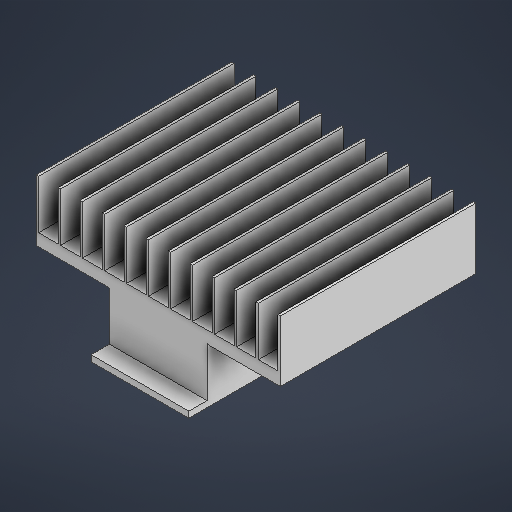
# Autodesk Inventor part: Heatsink_and_Amplifier
Saved by Autodesk Inventor 2026.2 (Build 302298010, 298A)
## iProperties
Created: 2026-09-21
Part Number: Heatsink_and_Amplifier
Material: Generic
Document SubType Name: Modeling
Designer: aiden
Density: 1 g/cm^3
Appearance: Default
Author: aiden
Autodesk Inventor part; units mm, degrees
ref_plane "YZ Plane" through (0, 0, 0) normal (1, 0, 0) x (0, 1, 0)
ref_plane "XZ Plane" through (0, 0, 0) normal (0, 1, 0) x (-1, 0, 0)
ref_plane "XY Plane" through (0, 0, 0) normal (0, 0, 1) x (1, 0, 0)
sketch "Sketch1" plane through (0, 0, 0) normal (0, 1, 0) x (-1, 0, 0)
  line L0 (-63.5, -50.8) -> (63.5, -50.8)
  line L1 (63.5, -50.8) -> (63.5, 50.8)
  line L2 (63.5, 50.8) -> (-63.5, 50.8)
  line L3 (-63.5, 50.8) -> (-63.5, -50.8)
  line L4 (-63.5, -50.8) -> (63.5, 50.8) construction
  line L5 (63.5, -50.8) -> (-63.5, 50.8) construction
  point P0 (0, 0)
  dimension "d0" = 127
  dimension "d1" = 101.6
  constraints: 12 end point, 2 midpoint, 2 parallel, 1 horizontal, 1 perpendicular
  measures "d0" distance of L2.end L1.end
  measures "d1" distance of L1.end L0.end
extrude "Extrusion1" add sketch "Sketch1" along normal blind 31.75
sketch "Sketch2" plane through (-63.5, 0, 50.8) normal (0, 0, 1) x (1, 0, 0)
  line L0 (0, 0) -> (127, 0) projected
  line L1 (0, 0) -> (0, 6.35)
  line L2 (0, 31.75) -> (127, 31.75) projected
  line L3 (0, 6.35) -> (127, 6.35) construction
  line L4 (127, 0) -> (0, 0)
  line L5 (0, 6.35) -> (0, 31.75)
  line L6 (0, 31.75) -> (1.27, 31.75)
  line L7 (1.27, 31.75) -> (1.27, 6.35)
  line L8 (1.27, 6.35) -> (0, 6.35)
  line L9 (127, 0) -> (127, 31.75) projected
  line L10 (127, 31.75) -> (127, 0)
  line L11 (11.43, 6.35) -> (11.43, 31.75)
  line L12 (11.43, 31.75) -> (12.7, 31.75)
  line L13 (12.7, 31.75) -> (12.7, 6.35)
  line L14 (12.7, 6.35) -> (11.43, 6.35)
  line L15 (22.86, 6.35) -> (22.86, 31.75)
  line L16 (22.86, 31.75) -> (24.13, 31.75)
  line L17 (24.13, 31.75) -> (24.13, 6.35)
  line L18 (24.13, 6.35) -> (22.86, 6.35)
  line L19 (34.29, 6.35) -> (34.29, 31.75)
  line L20 (34.29, 31.75) -> (35.56, 31.75)
  line L21 (35.56, 31.75) -> (35.56, 6.35)
  line L22 (35.56, 6.35) -> (34.29, 6.35)
  line L23 (45.72, 6.35) -> (45.72, 31.75)
  line L24 (45.72, 31.75) -> (46.99, 31.75)
  line L25 (46.99, 31.75) -> (46.99, 6.35)
  line L26 (46.99, 6.35) -> (45.72, 6.35)
  line L27 (57.15, 6.35) -> (57.15, 31.75)
  line L28 (57.15, 31.75) -> (58.42, 31.75)
  line L29 (58.42, 31.75) -> (58.42, 6.35)
  line L30 (58.42, 6.35) -> (57.15, 6.35)
  line L31 (68.58, 6.35) -> (68.58, 31.75)
  line L32 (68.58, 31.75) -> (69.85, 31.75)
  line L33 (69.85, 31.75) -> (69.85, 6.35)
  line L34 (69.85, 6.35) -> (68.58, 6.35)
  line L35 (80.01, 6.35) -> (80.01, 31.75)
  line L36 (80.01, 31.75) -> (81.28, 31.75)
  line L37 (81.28, 31.75) -> (81.28, 6.35)
  line L38 (81.28, 6.35) -> (80.01, 6.35)
  line L39 (91.44, 6.35) -> (91.44, 31.75)
  line L40 (91.44, 31.75) -> (92.71, 31.75)
  line L41 (92.71, 31.75) -> (92.71, 6.35)
  line L42 (92.71, 6.35) -> (91.44, 6.35)
  line L43 (102.87, 6.35) -> (102.87, 31.75)
  line L44 (102.87, 31.75) -> (104.14, 31.75)
  line L45 (104.14, 31.75) -> (104.14, 6.35)
  line L46 (104.14, 6.35) -> (102.87, 6.35)
  line L47 (114.3, 6.35) -> (114.3, 31.75)
  line L48 (114.3, 31.75) -> (115.57, 31.75)
  line L49 (115.57, 31.75) -> (115.57, 6.35)
  line L50 (115.57, 6.35) -> (114.3, 6.35)
  line L51 (125.73, 6.35) -> (125.73, 31.75)
  line L52 (125.73, 31.75) -> (127, 31.75)
  line L53 (127, 31.75) -> (127, 6.35)
  line L54 (127, 6.35) -> (125.73, 6.35)
  line L55 (0, 31.75) -> (127, 31.75)
  line L56 (127, 31.75) -> (127, 6.35)
  line L57 (127, 6.35) -> (0, 6.35)
  line L58 (0, 6.35) -> (0, 31.75)
  point P0 (0.635, 31.75)
  point P1 (12.065, 31.75)
  point P2 (23.495, 31.75)
  point P3 (34.925, 31.75)
  point P4 (46.355, 31.75)
  point P5 (57.785, 31.75)
  point P6 (69.215, 31.75)
  point P7 (80.645, 31.75)
  point P8 (92.075, 31.75)
  point P9 (103.505, 31.75)
  point P10 (114.935, 31.75)
  point P11 (126.365, 31.75)
  point P12 (126.365, 31.75)
  point P13 (125.73, 6.35)
  point P14 (115.57, 31.75)
  point P15 (104.14, 6.35)
  point P16 (114.3, 6.35)
  point P17 (114.3, 31.75)
  point P18 (104.14, 31.75)
  point P19 (92.71, 6.35)
  point P20 (102.87, 6.35)
  point P21 (102.87, 31.75)
  point P22 (92.71, 31.75)
  point P23 (81.28, 6.35)
  point P24 (91.44, 6.35)
  point P25 (91.44, 31.75)
  point P26 (81.28, 31.75)
  point P27 (80.01, 6.35)
  point P28 (80.01, 31.75)
  point P29 (69.85, 31.75)
  point P30 (58.42, 6.35)
  point P31 (68.58, 6.35)
  point P32 (68.58, 31.75)
  point P33 (58.42, 31.75)
  point P34 (57.15, 6.35)
  point P35 (57.15, 31.75)
  point P36 (46.99, 31.75)
  point P37 (35.56, 6.35)
  point P38 (45.72, 6.35)
  point P39 (45.72, 31.75)
  point P40 (35.56, 31.75)
  point P41 (24.13, 6.35)
  point P42 (34.29, 31.75)
  point P43 (24.13, 31.75)
  point P44 (12.7, 6.35)
  point P45 (22.86, 31.75)
  point P46 (12.7, 31.75)
  point P47 (11.43, 31.75)
  point P48 (1.27, 31.75)
  dimension "d4" = 6.35
  dimension "d5" = 1.27
  dimension "d36" = 11.43
  dimension "d41" = 0.635
  constraints: 110 end point, 4 perpendicular, 3 horizontal, 2 collinear, 2 midpoint, 2 point on line, 1 parallel, 1 vertical, 103 other
  measures "d4" distance of L0.start L1.end
  measures "d5" distance between parallel lines of L5 L7
  measures "d36" distance of L1.end L11.start
  measures "d41" distance of L9.end point (126.365, 31.75)
extrude "Extrusion2" cut sketch "Sketch2" against normal blind 122.2375 contours L7 L2 L11 L57 | L57 L49 L2 L51 | L13 L2 L15 L57 | L57 L45 L2 L47 | L17 L2 L19 L57 | L57 L41 L2 L43 | L21 L2 L23 L57 | L57 L37 L2 L39 | L25 L2 L27 L57 | L57 L33 L2 L35 | L29 L2 L31 L57
sketch "Sketch3" plane through (0, 0, 0) normal (0, -1, 0) x (1, 0, 0)
  line L0 (25.4, -60.325) -> (-25.4, -60.325)
  line L1 (-25.4, -60.325) -> (-25.4, 60.325)
  line L2 (-25.4, 60.325) -> (25.4, 60.325)
  line L3 (25.4, 60.325) -> (25.4, -60.325)
  line L4 (25.4, -60.325) -> (-25.4, 60.325) construction
  line L5 (-25.4, -60.325) -> (25.4, 60.325) construction
  point P0 (0, 0)
  dimension "d44" = 50.8
  dimension "d45" = 120.65
  constraints: 12 end point, 2 midpoint, 2 parallel, 1 horizontal, 1 perpendicular
  measures "d44" distance of L1.end L2.end
  measures "d45" distance of L0.end L1.end
extrude "Extrusion3" add sketch "Sketch3" along normal blind 28.575
sketch "Sketch4" plane through (0, 0, 0) normal (0, 1, 0) x (1, 0, 0)
  line L0 (25.4, 50.8) -> (-25.4, 50.8) projected
  line L1 (25.4, 60.325) -> (25.4, 50.8) projected
  line L2 (-25.4, 60.325) -> (25.4, 60.325) projected
  line L3 (-25.4, 50.8) -> (-25.4, 60.325) projected
  line L4 (-25.4, -50.8) -> (25.4, -50.8) projected
  line L5 (-25.4, -60.325) -> (-25.4, -50.8) projected
  line L6 (25.4, -60.325) -> (-25.4, -60.325) projected
  line L7 (25.4, -50.8) -> (25.4, -60.325) projected
  line L8 (-25.4, -60.325) -> (-25.4, 60.325) projected
  line L9 (-25.4, 60.325) -> (25.4, 60.325)
  line L10 (25.4, 60.325) -> (25.4, 50.8)
  line L11 (25.4, 50.8) -> (-25.4, 50.8)
  line L12 (-25.4, 50.8) -> (-25.4, 60.325)
  line L13 (-25.4, -50.8) -> (25.4, -50.8)
  line L14 (25.4, -50.8) -> (25.4, -60.325)
  line L15 (25.4, -60.325) -> (-25.4, -60.325)
  line L16 (-25.4, -60.325) -> (-25.4, -50.8)
  point P0 (0, 0)
  constraints: 16 end point, 4 parallel, 2 horizontal, 2 perpendicular
extrude "Extrusion4" cut sketch "Sketch4" against normal blind 25.4
body "Solid1"
